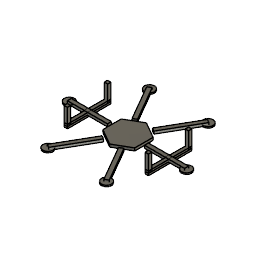
HexacopterFrame(OctoFly) (Autodesk Fusion 360 design; units mm, degrees)
part number: 2026-05-07-23-01-08-610
Autodesk Fusion 360 part; units mm, degrees
sketch "Sketch1" plane through (0, 0, 0) normal (0, 0, 1) x (1, 0, 0)
  line L0 (47.6314, 27.5) -> (0, 55)
  line L1 (0, 55) -> (-47.6314, 27.5)
  line L2 (-47.6314, 27.5) -> (-47.6314, -27.5)
  line L3 (-47.6314, -27.5) -> (0, -55)
  line L4 (0, -55) -> (47.6314, -27.5)
  line L5 (47.6314, -27.5) -> (47.6314, 27.5)
extrude "Extrude1" add sketch "Sketch1" along normal blind 8 makes body 1
sketch "Sketch2" plane through (0, 0, 0) normal (0, 0, 1) x (1, 0, 0)
  line L0 (55, 6) -> (55, -6)
  line L1 (55, -6) -> (175, -6)
  line L2 (175, -6) -> (175, 6)
  line L3 (175, 6) -> (55, 6)
extrude "Extrude2" add sketch "Sketch2" along normal blind 8 separate body makes body 2
sketch "Sketch3" plane through (0, 0, 0) normal (0, 0, 1) x (1, 0, 0)
  circle A0 centre (175, 0) radius 15
extrude "Extrude3" add sketch "Sketch3" along normal blind 4 separate body makes body 3
sketch "Sketch4" plane through (0, 0, 0) normal (0, 0, 1) x (1, 0, 0)
  line L0 (22.3038, 50.6314) -> (32.6962, 44.6314)
  line L1 (32.6962, 44.6314) -> (92.6962, 148.5544)
  line L2 (92.6962, 148.5544) -> (82.3038, 154.5544)
  line L3 (82.3038, 154.5544) -> (22.3038, 50.6314)
extrude "Extrude4" add sketch "Sketch4" along normal blind 8 separate body makes body 4
sketch "Sketch5" plane through (0, 0, 0) normal (0, 0, 1) x (1, 0, 0)
  circle A0 centre (87.5, 151.5544) radius 15
extrude "Extrude5" add sketch "Sketch5" along normal blind 4 separate body makes body 5
sketch "Sketch6" plane through (0, 0, 0) normal (0, 0, 1) x (1, 0, 0)
  line L0 (-32.6962, 44.6314) -> (-22.3038, 50.6314)
  line L1 (-22.3038, 50.6314) -> (-82.3038, 154.5544)
  line L2 (-82.3038, 154.5544) -> (-92.6962, 148.5544)
  line L3 (-92.6962, 148.5544) -> (-32.6962, 44.6314)
extrude "Extrude6" add sketch "Sketch6" along normal blind 8 separate body makes body 6
sketch "Sketch7" plane through (0, 0, 0) normal (0, 0, 1) x (1, 0, 0)
  circle A0 centre (-87.5, 151.5544) radius 15
extrude "Extrude7" add sketch "Sketch7" along normal blind 4 separate body makes body 7
sketch "Sketch8" plane through (0, 0, 0) normal (0, 0, 1) x (1, 0, 0)
  line L0 (-55, -6) -> (-55, 6)
  line L1 (-55, 6) -> (-175, 6)
  line L2 (-175, 6) -> (-175, -6)
  line L3 (-175, -6) -> (-55, -6)
extrude "Extrude8" add sketch "Sketch8" along normal blind 8 separate body makes body 8
sketch "Sketch9" plane through (0, 0, 0) normal (0, 0, 1) x (1, 0, 0)
  circle A0 centre (-175, 0) radius 15
extrude "Extrude9" add sketch "Sketch9" along normal blind 4 separate body makes body 9
sketch "Sketch10" plane through (0, 0, 0) normal (0, 0, 1) x (1, 0, 0)
  line L0 (-22.3038, -50.6314) -> (-32.6962, -44.6314)
  line L1 (-32.6962, -44.6314) -> (-92.6962, -148.5544)
  line L2 (-92.6962, -148.5544) -> (-82.3038, -154.5544)
  line L3 (-82.3038, -154.5544) -> (-22.3038, -50.6314)
extrude "Extrude10" add sketch "Sketch10" along normal blind 8 separate body makes body 10
sketch "Sketch11" plane through (0, 0, 0) normal (0, 0, 1) x (1, 0, 0)
  circle A0 centre (-87.5, -151.5544) radius 15
extrude "Extrude11" add sketch "Sketch11" along normal blind 4 separate body makes body 11
sketch "Sketch12" plane through (0, 0, 0) normal (0, 0, 1) x (1, 0, 0)
  line L0 (32.6962, -44.6314) -> (22.3038, -50.6314)
  line L1 (22.3038, -50.6314) -> (82.3038, -154.5544)
  line L2 (82.3038, -154.5544) -> (92.6962, -148.5544)
  line L3 (92.6962, -148.5544) -> (32.6962, -44.6314)
extrude "Extrude12" add sketch "Sketch12" along normal blind 8 separate body makes body 12
sketch "Sketch13" plane through (0, 0, 0) normal (0, 0, 1) x (1, 0, 0)
  circle A0 centre (87.5, -151.5544) radius 15
extrude "Extrude13" add sketch "Sketch13" along normal blind 4 separate body makes body 13
sketch "Sketch14" plane through (0, 0, 0) normal (0, 0, 1) x (1, 0, 0)
  line L0 (-126, 55) -> (-116, 55)
  line L1 (-116, 55) -> (-116, 65)
  line L2 (-116, 65) -> (-126, 65)
  line L3 (-126, 65) -> (-126, 55)
extrude "Extrude14" add sketch "Sketch14" along normal blind 50 separate body makes body 14
sketch "Sketch15" plane through (0, 0, 0) normal (0, 0, 1) x (1, 0, 0)
  line L0 (-126, -65) -> (-116, -65)
  line L1 (-116, -65) -> (-116, -55)
  line L2 (-116, -55) -> (-126, -55)
  line L3 (-126, -55) -> (-126, -65)
extrude "Extrude15" add sketch "Sketch15" along normal blind 50 separate body makes body 15
sketch "Sketch16" plane through (0, 0, 0) normal (0, 0, 1) x (1, 0, 0)
  line L0 (-126, -65) -> (-116, -65)
  line L1 (-116, -65) -> (-116, 65)
  line L2 (-116, 65) -> (-126, 65)
  line L3 (-126, 65) -> (-126, -65)
extrude "Extrude16" add sketch "Sketch16" along normal mid plane 12 separate body makes body 16
sketch "Sketch17" plane through (0, 0, 0) normal (0, 0, 1) x (1, 0, 0)
  line L0 (-126, -60) -> (-116, -60)
  line L1 (-116, -60) -> (-116, 60)
  line L2 (-116, 60) -> (-126, 60)
  line L3 (-126, 60) -> (-126, -60)
extrude "Extrude17" add sketch "Sketch17" along normal blind 6 separate body makes body 17
sketch "Sketch18" plane through (0, 0, 0) normal (0, 0, 1) x (1, 0, 0)
  line L0 (116, 55) -> (126, 55)
  line L1 (126, 55) -> (126, 65)
  line L2 (126, 65) -> (116, 65)
  line L3 (116, 65) -> (116, 55)
extrude "Extrude18" add sketch "Sketch18" along normal blind 50 separate body makes body 18
sketch "Sketch19" plane through (0, 0, 0) normal (0, 0, 1) x (1, 0, 0)
  line L0 (116, -65) -> (126, -65)
  line L1 (126, -65) -> (126, -55)
  line L2 (126, -55) -> (116, -55)
  line L3 (116, -55) -> (116, -65)
extrude "Extrude19" add sketch "Sketch19" along normal blind 50 separate body makes body 19
sketch "Sketch20" plane through (0, 0, 0) normal (0, 0, 1) x (1, 0, 0)
  line L0 (116, -65) -> (126, -65)
  line L1 (126, -65) -> (126, 65)
  line L2 (126, 65) -> (116, 65)
  line L3 (116, 65) -> (116, -65)
extrude "Extrude20" add sketch "Sketch20" along normal mid plane 12 separate body makes body 20
sketch "Sketch21" plane through (0, 0, 0) normal (0, 0, 1) x (1, 0, 0)
  line L0 (116, -60) -> (126, -60)
  line L1 (126, -60) -> (126, 60)
  line L2 (126, 60) -> (116, 60)
  line L3 (116, 60) -> (116, -60)
extrude "Extrude21" add sketch "Sketch21" along normal blind 6 separate body makes body 21
